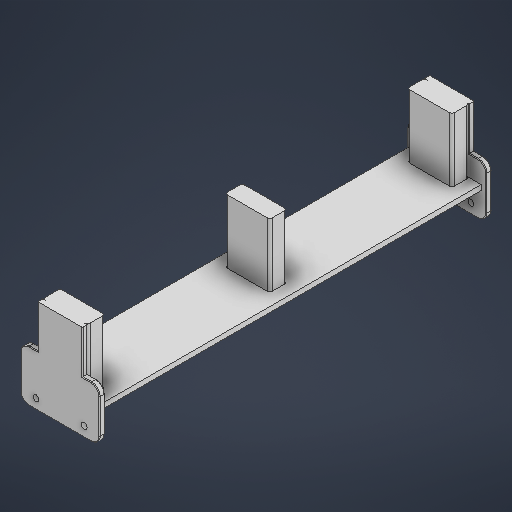
# Autodesk Inventor part: SACMI D-PA UPPER FRAME
Saved by Autodesk Inventor 2025 (Build 290162000, 162)
## iProperties
Created: 2024-05-20
Part Number: SACMI D-PA UPPER FRAME
Material: Generic
Document SubType Name: Modeling
Designer: zulet
Density: 1 g/cm^3
Appearance: Default
Author: zulet
Autodesk Inventor part; units mm, degrees
ref_plane "YZ Plane" through (0, 0, 0) normal (1, 0, 0) x (0, 1, 0)
ref_plane "XZ Plane" through (0, 0, 0) normal (0, 1, 0) x (-1, 0, 0)
ref_plane "XY Plane" through (0, 0, 0) normal (0, 0, 1) x (1, 0, 0)
sketch "Sketch1" plane through (0, 0, 0) normal (0, 1, 0) x (-1, 0, 0)
  line L0 (115, 50) -> (-115, 50)
  line L1 (-130, 35) -> (-130, -35)
  line L2 (-115, -50) -> (115, -50)
  line L3 (130, -35) -> (130, 35)
  line L4 (130, 50) -> (-130, -50) construction
  line L5 (-130, 50) -> (130, -50) construction
  arc A0 (115, -50) -> (130, -35) centre (115, -35) ccw
  arc A1 (-130, -35) -> (-115, -50) centre (-115, -35) ccw
  arc A2 (-115, 50) -> (-130, 35) centre (-115, 35) ccw
  arc A3 (130, 35) -> (115, 50) centre (115, 35) ccw
  line L6 (115, -42) -> (-115, -42)
  arc A4 (-122, -35) -> (-115, -42) centre (-115, -35) ccw
  line L7 (-122, -35) -> (-122, 35)
  arc A5 (-115, 42) -> (-122, 35) centre (-115, 35) ccw
  line L8 (-115, 42) -> (115, 42)
  arc A6 (122, 35) -> (115, 42) centre (115, 35) ccw
  line L9 (122, 35) -> (122, -35)
  arc A7 (115, -42) -> (122, -35) centre (115, -35) ccw
  line L10 (0, 1060) -> (0, -1060) construction
  arc A8 (-130, -1095) -> (-115, -1110) centre (-115, -1095) ccw
  arc A9 (-122, -1095) -> (-115, -1102) centre (-115, -1095) ccw
  line L11 (-130, -1025) -> (-130, -1095)
  line L12 (-122, -1095) -> (-122, -1025)
  line L13 (115, -1102) -> (-115, -1102)
  line L14 (115, -1010) -> (-115, -1010)
  line L15 (-115, -1110) -> (115, -1110)
  line L16 (122, -1025) -> (122, -1095)
  arc A10 (115, -1102) -> (122, -1095) centre (115, -1095) ccw
  arc A11 (115, -1110) -> (130, -1095) centre (115, -1095) ccw
  line L17 (130, -1095) -> (130, -1025)
  line L18 (-130, -1010) -> (130, -1110) construction
  line L19 (130, -1010) -> (-130, -1110) construction
  line L20 (-115, -1018) -> (115, -1018)
  arc A12 (-115, -1018) -> (-122, -1025) centre (-115, -1025) ccw
  arc A13 (-115, -1010) -> (-130, -1025) centre (-115, -1025) ccw
  arc A14 (122, -1025) -> (115, -1018) centre (115, -1025) ccw
  arc A15 (130, -1025) -> (115, -1010) centre (115, -1025) ccw
  arc A16 (-130, 1025) -> (-115, 1010) centre (-115, 1025) ccw
  arc A17 (-122, 1025) -> (-115, 1018) centre (-115, 1025) ccw
  line L21 (-130, 1095) -> (-130, 1025)
  line L22 (-122, 1025) -> (-122, 1095)
  line L23 (115, 1018) -> (-115, 1018)
  line L24 (115, 1110) -> (-115, 1110)
  line L25 (-115, 1010) -> (115, 1010)
  line L26 (122, 1095) -> (122, 1025)
  arc A18 (115, 1018) -> (122, 1025) centre (115, 1025) ccw
  arc A19 (115, 1010) -> (130, 1025) centre (115, 1025) ccw
  line L27 (130, 1025) -> (130, 1095)
  line L28 (-130, 1110) -> (130, 1010) construction
  line L29 (130, 1110) -> (-130, 1010) construction
  line L30 (-115, 1102) -> (115, 1102)
  arc A20 (-115, 1102) -> (-122, 1095) centre (-115, 1095) ccw
  arc A21 (-115, 1110) -> (-130, 1095) centre (-115, 1095) ccw
  arc A22 (122, 1095) -> (115, 1102) centre (115, 1095) ccw
  arc A23 (130, 1095) -> (115, 1110) centre (115, 1095) ccw
  line L31 (-200, 1110) -> (200, 1110)
  line L32 (200, 1110) -> (200, -1110)
  line L33 (200, -1110) -> (-200, -1110)
  line L34 (-200, -1110) -> (-200, 1110)
  line L35 (-200, 1110) -> (200, -1110) construction
  line L36 (200, 1110) -> (-200, -1110) construction
  point P0 (0, 0)
  point P1 (0, -1060)
  point P2 (0, 1060)
  point P3 (115, -1110)
  point P4 (115, 1110)
  point P5 (-115, 1110)
  point P6 (-115, -1110)
  dimension "d0" = 260
  dimension "d1" = 100
  dimension "d2" = 15
  dimension "d3" = 8
  dimension "d4" = 2120
  dimension "d7" = 1060
  dimension "d12" = 400
  constraints: 74 end point, 48 point on circle, 24 centre point, 24 point on line, 8 tangent, 6 parallel, 5 midpoint, 3 equal radius, 3 perpendicular, 2 horizontal, 2 vertical, 1 collinear, 93 other
  measures "d0" distance of L5.end L4.end
  measures "d1" distance of L4.end L5.start
  measures "d2" radius of A0
  measures "d3" distance between parallel lines of L2 L6
  measures "d4" distance of L10.start L10.end
  measures "d7" distance of A1.centre A8.centre
  measures "d12" distance of L32.end L33.end
extrude "Extrusion1" add sketch "Sketch1" along normal blind 370 contours A3 L3 A0 L2 A1 L1 A2 L0 | L11 A13 L14 A15 L17 A11 L15 A8 | L24 A23 L27 A19 L25 A16 L21 A21
extrude "Extrusion2" add sketch "Sketch1" against normal blind 30 contours A3 L3 A0 L2 A1 L1 A2 L0 | L6 A4 L7 A5 L8 A6 L9 A7 | L11 A13 L14 A15 L17 A11 L15 A8 | A8 L33 L34 L31 A21 L21 A16 L25 A19 L27 A23 L32 A11 L17 A15 L14 A13 L11 | L24 A23 L27 A19 L25 A16 L21 A21 | L12 A12 L20 A14 L16 A10 L13 A9 | L22 A20 L30 A22 L26 A18 L23 A17
sketch "Sketch2" plane through (-115, 370, 1110) normal (0, 0, 1) x (1, 0, 0)
  line L0 (-15, -370) -> (-15, 0) construction
  line L1 (0, 0) -> (230, 0) projected
  line L2 (0, 0) -> (-15, 0) projected
  line L3 (245, 0) -> (230, 0) projected
  line L4 (245, -370) -> (245, 0) construction
  line L5 (295, -550) -> (-65, -550)
  line L6 (-115, -500) -> (-115, -300)
  line L7 (345, -300) -> (345, -500)
  line L8 (345, -550) -> (-115, -250) construction
  line L9 (-115, -550) -> (345, -250) construction
  line L10 (-85, -370) -> (-85, -400) construction
  line L11 (315, -370) -> (315, -400) construction
  line L12 (-15, 0) -> (-15, -250)
  line L13 (245, 0) -> (245, -250)
  line L14 (-65, -250) -> (-15, -250)
  line L15 (245, -250) -> (295, -250)
  line L16 (315, -400) -> (-85, -400) construction
  arc A0 (-65, -250) -> (-115, -300) centre (-65, -300) ccw
  arc A1 (-115, -500) -> (-65, -550) centre (-65, -500) ccw
  arc A2 (295, -550) -> (345, -500) centre (295, -500) ccw
  arc A3 (345, -300) -> (295, -250) centre (295, -300) ccw
  circle A4 centre (-25, -491) radius 17.5
  line L17 (115, -400) -> (115, -550) construction
  circle A5 centre (255, -491) radius 17.5
  point P0 (115, -370)
  point P1 (115, -400)
  point P2 (-15, -200)
  point P3 (245, -200)
  dimension "d18" = 150
  dimension "d19" = 150
  dimension "d20" = 50
  dimension "d21" = 35
  dimension "d23" = 140
  dimension "d47" = 30
  dimension "d48" = 30
  dimension "d49" = 91
  constraints: 20 end point, 10 point on line, 8 point on circle, 8 tangent, 6 centre point, 4 midpoint, 3 equal radius, 3 parallel, 1 horizontal, 1 perpendicular, 1 symmetric about line, 1 other
  measures "d18" distance between parallel lines of L16 L14
  measures "d19" distance between parallel lines of L16 L5
  measures "d20" radius of A0
  measures "d21" diameter of A4
  measures "d23" horizontal distance of point (115, -400) A4.centre
  measures "d47" distance between parallel lines of L6 L10
  measures "d48" distance between parallel lines of L11 L7
  measures "d49" distance from line of L16 A4.centre
extrude "Extrusion3" add sketch "Sketch2" along normal blind 30
fillet "Fillet1" radius 4 18 edges at (130, 245, 1110) (130, 245, 1140) (-130, 245, 1110) (-130, 245, 1140) (-230, -30, 1110) (-215.3553, 105.3553, 1110) (-230, -30, 1140) (-215.3553, -165.3553, 1140) (0, -180, 1140) (215.3553, -165.3553, 1140) (230, -30, 1140) (215.3553, 105.3553, 1140) (-215.3553, 105.3553, 1140) (-215.3553, -165.3553, 1110) (0, -180, 1110) (215.3553, -165.3553, 1110) (230, -30, 1110) (215.3553, 105.3553, 1110)
mirror "Mirror1" about plane through (0, 0, 0) normal (0, 0, 1) of "Extrusion3", "Fillet1"
sketch "Sketch3" plane through (0, -30, 0) normal (0, -1, 0) x (1, 0, 0)
  line L0 (-115, 1110) -> (-126, 1110) construction
  line L1 (200, 1110) -> (-200, 1110) construction
  line L2 (0, 1110) -> (0, -1110) construction
  line L3 (-200, -1110) -> (200, -1110) construction
  point P0 (0, 0)
  point P1 (-140, 1080)
  point P2 (181, 1110)
  point P3 (-181, 1110)
  point P4 (-181, -1110)
  point P5 (181, -1110)
  point P6 (-140, 1020)
  point P7 (-140, 960)
  point P8 (-140, 900)
  point P9 (-140, 840)
  point P10 (-140, 780)
  point P11 (-140, 720)
  point P12 (-140, 660)
  point P13 (-140, 600)
  point P14 (-140, 540)
  point P15 (-140, 480)
  point P16 (-140, 420)
  point P17 (-140, 360)
  point P18 (-140, 300)
  point P19 (-140, 240)
  point P20 (-140, 180)
  point P21 (-140, 120)
  point P22 (-140, 60)
  point P23 (-140, 0)
  point P24 (-140, -60)
  point P25 (-140, -120)
  point P26 (-140, -180)
  point P27 (-140, -240)
  point P28 (-140, -300)
  point P29 (-140, -360)
  point P30 (-140, -420)
  point P31 (-140, -480)
  point P32 (-140, -540)
  point P33 (-140, -600)
  point P34 (-140, -660)
  point P35 (-140, -720)
  point P36 (-140, -780)
  point P37 (-140, -840)
  point P38 (-140, -900)
  point P39 (-140, -960)
  point P40 (-140, -1020)
  point P41 (-140, -1080)
  point P42 (140, 1080)
  point P43 (140, 1020)
  point P44 (140, 960)
  point P45 (140, 900)
  point P46 (140, 840)
  point P47 (140, 780)
  point P48 (140, 720)
  point P49 (140, 660)
  point P50 (140, 600)
  point P51 (140, 540)
  point P52 (140, 480)
  point P53 (140, 420)
  point P54 (140, 360)
  point P55 (140, 300)
  point P56 (140, 240)
  point P57 (140, 180)
  point P58 (140, 120)
  point P59 (140, 60)
  point P60 (140, 0)
  point P61 (140, -60)
  point P62 (140, -120)
  point P63 (140, -180)
  point P64 (140, -240)
  point P65 (140, -300)
  point P66 (140, -360)
  point P67 (140, -420)
  point P68 (140, -480)
  point P69 (140, -540)
  point P70 (140, -600)
  point P71 (140, -660)
  point P72 (140, -720)
  point P73 (140, -780)
  point P74 (140, -840)
  point P75 (140, -900)
  point P76 (140, -960)
  point P77 (140, -1020)
  point P78 (140, -1080)
  dimension "d27" = 30
  dimension "d28" = 140
  dimension "d29" = 2220
  dimension "d32" = 60
  dimension "d35" = 280
  constraints: 2 end point, 2 midpoint, 1 horizontal, 1 vertical, 73 other
  measures "d27" distance from line of L0 point (-140, 1080)
  measures "d28" distance from line of L2 point (-140, 1080)
  measures "d29" distance of L2.start L2.end
  measures "d32" distance of point (-140, 1080) point (-140, 1020)
  measures "d35" distance of point (-140, 1080) point (140, 1080)
hole "Hole1" at (-140, -30, 1080) at (-140, -30, 1020) at (-140, -30, 960) at (-140, -30, 900) at (-140, -30, 840) at (-140, -30, 780) at (-140, -30, 720) at (-140, -30, 660) at (-140, -30, 600) at (-140, -30, 540) at (-140, -30, 480) at (-140, -30, 420) at (-140, -30, 360) at (-140, -30, 300) at (-140, -30, 240) at (-140, -30, 180) at (-140, -30, 120) at (-140, -30, 60) at (-140, -30, 0) at (-140, -30, -60) at (-140, -30, -120) at (-140, -30, -180) at (-140, -30, -240) at (-140, -30, -300) at (-140, -30, -360) at (-140, -30, -420) at (-140, -30, -480) at (-140, -30, -540) at (-140, -30, -600) at (-140, -30, -660) at (-140, -30, -720) at (-140, -30, -780) at (-140, -30, -840) at (-140, -30, -900) at (-140, -30, -960) at (-140, -30, -1020) at (-140, -30, -1080) at (140, -30, 1080) at (140, -30, 1020) at (140, -30, 960) at (140, -30, 900) at (140, -30, 840) at (140, -30, 780) at (140, -30, 720) at (140, -30, 660) at (140, -30, 600) at (140, -30, 540) at (140, -30, 480) at (140, -30, 420) at (140, -30, 360) direction (0, 1, 0) diameter 8 depth 15 and at (140, -30, 300) (140, -30, 240) (140, -30, 180) (140, -30, 120) (140, -30, 60) (140, -30, 0) (140, -30, -60) (140, -30, -120) (140, -30, -180) (140, -30, -240) (140, -30, -300) (140, -30, -360) (140, -30, -420) (140, -30, -480) (140, -30, -540) (140, -30, -600) (140, -30, -660) (140, -30, -720) (140, -30, -780) (140, -30, -840) (140, -30, -900) (140, -30, -960) (140, -30, -1020) (140, -30, -1080)
sketch "Sketch4" plane through (0, 370, 0) normal (0, 1, 0) x (1, 0, 0)
  line L0 (115, -42) -> (-115, -42) projected
  arc A0 (-122, -35) -> (-115, -42) centre (-115, -35) ccw projected
  line L1 (115, -42) -> (-115, -42) projected
  arc A1 (115, -42) -> (122, -35) centre (115, -35) ccw projected
  line L2 (122, 35) -> (122, -35) projected
  arc A2 (122, 35) -> (115, 42) centre (115, 35) ccw projected
  line L3 (-115, 42) -> (115, 42) projected
  arc A3 (-115, 42) -> (-122, 35) centre (-115, 35) ccw projected
  line L4 (-122, -35) -> (-122, 35) projected
  arc A4 (115, 1018) -> (122, 1025) centre (115, 1025) ccw projected
  line L5 (122, 1095) -> (122, 1025) projected
  arc A5 (122, 1095) -> (115, 1102) centre (115, 1095) ccw projected
  line L6 (-115, 1102) -> (115, 1102) projected
  arc A6 (-115, 1102) -> (-122, 1095) centre (-115, 1095) ccw projected
  line L7 (-122, 1025) -> (-122, 1095) projected
  arc A7 (-122, 1025) -> (-115, 1018) centre (-115, 1025) ccw projected
  line L8 (115, 1018) -> (-115, 1018) projected
  arc A8 (115, -1102) -> (122, -1095) centre (115, -1095) ccw projected
  line L9 (122, -1025) -> (122, -1095) projected
  arc A9 (122, -1025) -> (115, -1018) centre (115, -1025) ccw projected
  line L10 (-115, -1018) -> (115, -1018) projected
  arc A10 (-115, -1018) -> (-122, -1025) centre (-115, -1025) ccw projected
  line L11 (-122, -1095) -> (-122, -1025) projected
  arc A11 (-122, -1095) -> (-115, -1102) centre (-115, -1095) ccw projected
  line L12 (115, -1102) -> (-115, -1102) projected
  point P0 (0, 0)
extrude "Extrusion4" add sketch "Sketch4" against normal blind 10
equation "\"d7\" = 0.5 * d4"
equation "\"d12\" = distanceBetweenRails + 2 * border"
equation "\"d14\" = height - plateThickness"
equation "\"d16\" = plateThickness"
equation "\"d23\" = 0.5 * distanceBetweenRails"
equation "\"d48\" = d47"
equation "\"d24\" = plateThickness"
equation "\"d28\" = 0.5 * distanceBetweenRails"
equation "\"d35\" = distanceBetweenRails"
equation "\"height\" = 400"
equation "\"plateThickness\" = 30"
equation "\"distanceBetweenRails\" = 280"
equation "\"border\" = 60"
body "Solid1"
